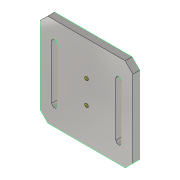
# Autodesk Inventor part: TL20240701-10200AT-004
Saved by Autodesk Inventor 2022.5 (Build 265521000, 521)
## iProperties
Category: ANTI BACK ASSY
Company: 현대트랜시스(대유)
Created: 2023-02-24
Part Number: TL20240701-10200AT-004
Checked By: 김형민
User Status: 1 x13
Material: SS400
Description: 0
Document SubType Name: Modeling
Mfg Approved By: 호상태
Designer: 백승윤
Stock Number: 004
Density: 7.85 g/cm^3
Appearance: Plating Zinc White
Project: SW-PJT
Engr Approved By: 김시현
DETAIL: Coveryor Assembly
M/C TITLE: CJ 제일제당 협동로봇 포장시스탬 PILOT 장비
PARTS NAME: MAIN PLATE
SPECIFICATION: TL20221201-080000C3-001
DocNumber: 221118_Standard_v1
Folder: .\
VDS_Category: 엔지니어링
Detail Description: Processed products
Title: BASE PLATE
Subject: SW차종 시트조립라인
Author: 백승윤
Revision Number: A
Autodesk Inventor part; units mm, degrees
ref_plane "YZ Plane" through (0, 0, 0) normal (1, 0, 0) x (0, 1, 0)
ref_plane "XZ Plane" through (0, 0, 0) normal (0, 1, 0) x (-1, 0, 0)
ref_plane "XY Plane" through (0, 0, 0) normal (0, 0, 1) x (1, 0, 0)
sketch "스케치9" plane through (0, 0, 0) normal (0, 0, 1) x (1, 0, 0)
  line L0 (-60, 60) -> (60, 60)
  line L1 (60, 60) -> (60, -60)
  line L2 (60, -60) -> (-60, -60)
  line L3 (-60, -60) -> (-60, 60)
  line L4 (-41.5, 35) -> (-41.5, -35) construction
  line L5 (-38, 35) -> (-38, -35)
  line L6 (-45, -35) -> (-45, 35)
  arc A0 (-38, 35) -> (-45, 35) centre (-41.5, 35) ccw
  arc A1 (-45, -35) -> (-38, -35) centre (-41.5, -35) ccw
  line L7 (41.5, 35) -> (41.5, -35) construction
  line L8 (45, 35) -> (45, -35)
  line L9 (38, -35) -> (38, 35)
  arc A2 (45, 35) -> (38, 35) centre (41.5, 35) ccw
  arc A3 (38, -35) -> (45, -35) centre (41.5, -35) ccw
  point P0 (0, 0)
  point P1 (-60, 0)
  point P2 (0, 60)
  point P3 (-41.5, 0)
  point P4 (41.5, 0)
  point P5 (-41.5, 0)
  point P6 (41.5, 0)
  dimension "d40" = 120
  dimension "d41" = 120
  dimension "d42" = 3.5
  dimension "d45" = 70
  dimension "d74" = 18.5
  dimension "d75" = 18.5
  dimension "d76" = 25
  constraints: 24 end point, 8 point on circle, 8 tangent, 5 parallel, 4 centre point, 4 midpoint, 3 horizontal alignment, 2 coincident, 2 vertical, 1 equal radius, 1 horizontal, 1 perpendicular, 1 vertical alignment
  measures "d40" distance of L0.start L0.end
  measures "d41" distance of L2.end L0.start
  measures "d42" radius of A0
  measures "d45" distance of L4.start L4.end
  measures "d74" distance between parallel lines of L4 L3
  measures "d75" distance between parallel lines of L1 L7
  measures "d76" distance from line of L0 L4.start
extrude "돌출4" add sketch "스케치9" along normal mid plane 9
sketch "스케치10" plane through (0, 0, 4.5) normal (0, 0, 1) x (1, 0, 0)
  line L0 (60, 60) -> (-60, 60) projected
  line L1 (-60, 60) -> (-60, -60) projected
  line L2 (60, -60) -> (60, 60) projected
  point P0 (0, 15)
  point P1 (0, -15)
  dimension "d66" = 30
  dimension "d70" = 120
  dimension "d71" = 60
  dimension "d72" = 45
  constraints: 1 vertical alignment
  measures "d66" distance of point (0, -15) point (0, 15)
  measures "d70" distance between parallel lines of L2 L1
  measures "d71" distance from line of point (0, 15) L2
  measures "d72" distance from line of L0 point (0, 15)
hole "구멍3" at (0, 15, 4.5) at (0, -15, 4.5) direction (0, 0, -1) diameter 4.917 end through all thread size "M6x1" class "6H" standard "TS profile"
chamfer "모따기1" distance 10 angle 45 4 edges at (60, 60, 0) (60, -60, 0) (-60, -60, 0) (-60, 60, 0)
equation "\"d71\" = 0.5 * d70"
